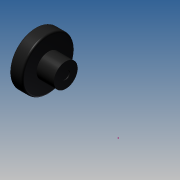
# Autodesk Inventor part: falsarueda
Saved by Autodesk Inventor 2011 (Build 150239000, 239)
## iProperties
Created: 2011-09-21
Part Number: falsarueda
Document SubType Name: Modeling
Designer: mgaspari
Density: 1 g/cm^3
Author: mgaspari
Autodesk Inventor part; units mm, degrees
ref_plane "YZ Plane" through (0, 0, 0) normal (1, 0, 0) x (0, 1, 0)
ref_plane "XZ Plane" through (0, 0, 0) normal (0, 1, 0) x (-1, 0, 0)
ref_plane "XY Plane" through (0, 0, 0) normal (0, 0, 1) x (1, 0, 0)
sketch "Sketch1" plane through (0, 0, 0) normal (0, 0, 1) x (1, 0, 0)
  point P0 (0, 0)
sketch "Sketch9" plane through (0, 0, 0) normal (0, 0, 1) x (1, 0, 0)
  line L0 (-12.03, 6.6772) -> (-12.03, 3.5022)
  line L1 (-13.62, 3.5022) -> (-13.62, 6.6772)
  line L2 (-12.05, 6.6772) -> (-13.62, 6.6772)
  line L3 (-13.62, 6.6772) -> (-12.03, 6.6772)
  line L4 (-13.62, 3.5022) -> (-12.03, 3.5022)
  point P0 (0, 0)
  dimension "d87" = 12.03
  dimension "d90" = 3.175
  constraints: 10 end point, 1 parallel, 1 vertical
  measures "d87" distance from line of point (0, 0) L0
  measures "d90" distance between parallel lines of L4 L2
revolve "Revolution1" add sketch "Sketch9" angle 360 about axis through (-13.62, 3.5022, 0) along (1, 0, 0)
sketch "Sketch10" plane through (-12.03, 3.5022, 0) normal (1, 0, 0) x (0, 0, -1)
  circle A0 centre (0.0724, 0) radius 1.45
  point P0 (0, -3.5022)
  constraints: 1 centre point
fillet "Fillet11" radius 0.2 2 edges at (-12.03, 0.3272, 0) (-13.62, 0.3272, 0)
extrude "Extrusion7" add sketch "Sketch10" along normal blind 2.1
sketch "Sketch12" plane through (-9.93, 3.5022, -0.0724) normal (1, 0, 0) x (0, 0, -1)
  circle A0 centre (0, 0) radius 1.45 projected
  circle A1 centre (0, 0) radius 0.5
  point P0 (-0.0724, -3.5022)
  constraints: 1 centre point, 1 coincident
extrude "Extrusion10" cut sketch "Sketch12" against normal blind 0.1 contours A1
body "Solid1"
